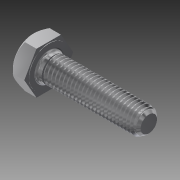
# Autodesk Inventor part: M10x40
Saved by Autodesk Inventor 2014 (Build 180170000, 170)
## iProperties
Created: 2013-10-10
Part Number: M10x40
Material: Srebrny
Document SubType Name: Modeling
Designer: Mikołaj
Density: 10.49 g/cm^3
Appearance: Srebrny
Author: Mikołaj
Autodesk Inventor part; units mm, degrees
ref_plane "YZ Plane" through (0, 0, 0) normal (1, 0, 0) x (0, 1, 0)
ref_plane "XZ Plane" through (0, 0, 0) normal (0, 1, 0) x (-1, 0, 0)
sketch "Szkic1" plane through (0, 0, 0) normal (1, 0, 0) x (0, 1, 0)
  line L0 (-4.9075, -8.5) -> (-9.815, 0)
  line L1 (-9.815, 0) -> (-4.9075, 8.5)
  line L2 (-4.9075, 8.5) -> (4.9075, 8.5)
  line L3 (4.9075, 8.5) -> (9.815, 0)
  line L4 (9.815, 0) -> (4.9075, -8.5)
  line L5 (4.9075, -8.5) -> (-4.9075, -8.5)
  point P0 (0, 0)
  point P1 (0, 0)
  dimension "d0" = 17
  constraints: 12 end point, 1 coincident, 13 other
  measures "d0" distance between parallel lines of L5 L2
extrude "Wyciągnięcie proste1" add sketch "Szkic1" along normal blind 6.3
sketch "Szkic2" plane through (6.3, 0, 0) normal (1, 0, 0) x (0, 0, -1)
  circle A0 centre (0, 0) radius 8
  dimension "d3" = 16
  constraints: 1 centre point, 1 coincident
  measures "d3" diameter of A0
extrude "Wyciągnięcie proste2" add sketch "Szkic2" along normal blind 0.2
ref_plane "Płaszczyzna konstrukcyjna1" through (0, -9.815, 0) normal (0, 0, 1) x (1, 0, 0)
sketch "Szkic3" plane through (0, -9.815, 0) normal (0, 0, 1) x (1, 0, 0)
  line L0 (0, 19.6299) -> (6.3, 19.6299) projected
  line L1 (0, 14.7224) -> (0, 19.6299) projected
  line L2 (0, 19.6299) -> (1.7, 19.6299)
  line L3 (0, 19.6299) -> (0, 17.9299)
  line L4 (0, 17.9299) -> (1.7, 19.6299)
  line L5 (0, 9.815) -> (6.9483, 9.815)
  dimension "d6" = 1.7
  dimension "d7" = 1.7
  constraints: 8 end point, 2 point on line, 1 perpendicular
  measures "d6" distance of L0.start L2.end
  measures "d7" distance of L0.start L3.end
revolve "Obrót1" cut sketch "Szkic3" angle 360 about axis through (0, 0, 0) along (1, 0, 0)
sketch "Szkic4" plane through (6.5, 0, 0) normal (1, 0, 0) x (0, 0, -1)
  circle A0 centre (0, 0) radius 8 projected
  circle A1 centre (0, 0) radius 4.188
  dimension "d9" = 8.376
  constraints: 1 centre point, 1 coincident
  measures "d9" diameter of A1
extrude "Wyciągnięcie proste3" add sketch "Szkic4" along normal blind 40 contours A1
sketch "Szkic5" plane through (0, -9.815, 0) normal (0, 0, 1) x (1, 0, 0)
  line L0 (6.5, 14.003) -> (6.5, 5.627) projected
  line L1 (6.5, 14.003) -> (46.5, 14.003) projected
  line L2 (6.5, 5.627) -> (46.5, 5.627) projected
  line L3 (6.5, 14.003) -> (7.7, 14.003)
  line L4 (7.7, 14.003) -> (7.7, 14.815)
  line L5 (7.25, 14.815) -> (7.7, 14.003)
  line L6 (7.25, 14.815) -> (6.95, 14.815)
  line L7 (6.95, 14.815) -> (6.5, 14.003)
  line L8 (-0.18, 9.815) -> (48.3952, 9.815)
  point P0 (0, 9.815)
  dimension "d12" = 1.2
  dimension "d14" = 0.45
  dimension "d15" = 0.3
  constraints: 12 end point, 1 parallel, 1 perpendicular, 1 point on line
  measures "d12" distance of L1.start L3.end
  measures "d14" distance of L4.end L5.start
  measures "d15" distance of L5.start L6.end
coil "Zwój1" sketch "Szkic5" operation add axis through (-0.18, 0, 0) along (1, 0, 0) pitch 1.5 turns 24.866667 hand right
sketch "Szkic6" plane through (6.5, 0, 0) normal (1, 0, 0) x (0, 0, -1)
  circle A0 centre (0, 0) radius 8 projected
  circle A1 centre (0, 0) radius 5
  point P0 (0, 4.188)
  dimension "d24" = 10
  constraints: 1 centre point, 1 coincident
  measures "d24" diameter of A1
extrude "Wyciągnięcie proste4" add sketch "Szkic6" along normal blind 2 contours A1
fillet "Zaokrąglenie1" radius 1 1 edges at (6.5, 0, 5)
sketch "Szkic7" plane through (43.8, 2.8023, -3.1123) normal (0, 0.7431448, 0.6691306) x (1, 0, 0)
  line L0 (1.2, 0) -> (0.75, 0.812) projected
  line L1 (0.75, 0.812) -> (0.45, 0.812) projected
  line L2 (0.45, 0.812) -> (0, 0) projected
  line L3 (1.2, 0) -> (0, 0) projected
  line L4 (0, 0) -> (1.2, 0)
  line L5 (0.75, 0.812) -> (1.2, 0)
  line L6 (0.75, 0.812) -> (0.45, 0.812)
  line L7 (0.45, 0.812) -> (0, 0)
  line L8 (-43.8, -4.188) -> (6.874, -4.188)
  constraints: 10 end point, 4 collinear, 1 parallel
coil "Zwój2" sketch "Szkic7" operation add axis through (0, 0, 0) along (1, 0, 0) pitch 1.5 turns 1 hand right taper -40
chamfer "Faza1" distance 0.9 angle 45 1 edges at (46.5, 0, 4.188)
